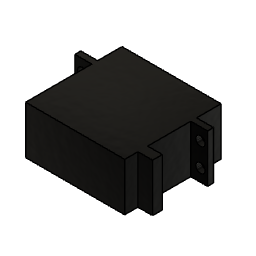
MG995 v10 (Autodesk Fusion 360 design; units mm, degrees)
Autodesk Fusion 360 part; units mm, degrees
sketch "Sketch1" plane through (0, 0, 0) normal (0, 1, 0) x (1, 0, 0)
  line L0 (0, 0) -> (40.47, 0)
  line L1 (40.47, 0) -> (40.47, -39.36)
  line L2 (40.47, -39.36) -> (0, -39.36)
  line L3 (0, -39.36) -> (0, 0)
  line L4 (40.47, -9.96) -> (47.35, -9.96)
  line L5 (47.35, -9.96) -> (47.35, -12.36)
  line L6 (47.35, -12.36) -> (40.47, -12.36)
  line L7 (40.47, -29.96) -> (46.47, -29.96)
  line L8 (46.47, -29.96) -> (46.47, -33.96)
  line L9 (46.47, -33.96) -> (40.47, -33.96)
  line L10 (20.235, 0) -> (20.235, -39.36) construction
  line L11 (0, -9.96) -> (-6.88, -9.96)
  line L12 (-6.88, -9.96) -> (-6.88, -12.36)
  line L13 (-6.88, -12.36) -> (0, -12.36)
  dimension "d1" = 40.47
  dimension "d2" = 39.36
  dimension "d3" = 6.88
  dimension "d4" = 2.4
  dimension "d5" = 27
  dimension "d6" = 6
  dimension "d7" = 4
  dimension "d8" = 5.4
  constraint horizontal L0
  constraint vertical L1
  constraint horizontal L2
  constraint vertical L3
  constraint coincident L0.start L3.end
  constraint coincident L1 L4.start
  constraint perpendicular L1 L4
  constraint perpendicular L4 L5
  constraint coincident L1 L6.end
  constraint perpendicular L1 L6
  constraint horizontal L7
  constraint coincident L1 L7.start
  constraint perpendicular L7 L8
  constraint coincident L1 L9.end
  constraint perpendicular L1 L9
  constraint midpoint L0 L10.start
  constraint midpoint L2 L10.end
  constraint symmetric L4.start L10 L11.start
  constraint symmetric L4.end L10 L11.end
  constraint symmetric L5.end L10 L12.end
  constraint symmetric L6.end L10 L13.end
  measures "d1" distance of L0.start L0.end
  measures "d2" distance of L0.start L2.end
  measures "d3" distance of L4.start L4.end
  measures "d4" distance of L4.end L5.end
  measures "d5" distance of L2 L6
  measures "d6" distance of L7.start L7.end
  measures "d7" distance of L7.end L8.end
  measures "d8" distance of L2 L9
extrude "Extrude1" add sketch "Sketch1" along normal blind 19.6
sketch "Sketch2" plane through (0, 0, 0) normal (0, 0, -1) x (-1, 0, 0)
  line L0 (-40.47, 0) -> (0, 0)
  line L1 (0, 0) -> (0, 19.6)
  line L2 (0, 19.6) -> (-40.47, 19.6)
  line L3 (-40.47, 19.6) -> (-40.47, 0)
  circle A0 centre (-30.8, 9.8) radius 2.92
  line L4 (0, 9.8) -> (-40.47, 9.8) construction
  dimension "d11" = 5.84
  dimension "d12" = 9.67
  constraint midpoint L1 L4.start
  constraint midpoint L3 L4.end
  constraint coincident A0.centre L4
  measures "d11" diameter of A0
  measures "d12" distance of L3 A0.centre
extrude "Extrude2" add sketch "Sketch2" along normal blind 3.81 contours A0
sketch "Sketch3" plane through (0, 0, 9.96) normal (0, 0, -1) x (-1, 0, 0)
  line L0 (-47.35, 0) -> (-40.47, 0)
  line L1 (-40.47, 0) -> (-40.47, 19.6)
  line L2 (-40.47, 19.6) -> (-47.35, 19.6)
  line L3 (-47.35, 19.6) -> (-47.35, 0)
  circle A0 centre (-44.425, 14.58) radius 1.915
  circle A1 centre (-44.425, 5.02) radius 1.915
  line L4 (-40.47, 9.8) -> (-47.35, 9.8) construction
  line L5 (-40.47, 0) -> (-40.47, 19.6)
  line L6 (0, 0) -> (0, 19.6)
  line L7 (0, 0) -> (-40.47, 0)
  line L8 (-40.47, 19.6) -> (0, 19.6)
  line L9 (-20.235, 19.6) -> (-20.235, 0) construction
  dimension "d15" = 3.83
  dimension "d16" = 3.83
  dimension "d17" = 9.56
  dimension "d19" = 2.925
  constraint midpoint L1 L4.start
  constraint midpoint L3 L4.end
  constraint symmetric A0 A1 L4
  constraint midpoint L8 L9.start
  constraint midpoint L7 L9.end
  measures "d15" diameter of A0
  measures "d16" diameter of A1
  measures "d17" distance of A0.centre A1.centre
  measures "d19" distance of L3 A0.centre
extrude "Extrude3" cut sketch "Sketch3" against normal up to surface (2.4 mm away) contours A0 | A1
ref_plane "WorkPlane1" through (20.235, 9.8, 4.98) normal (-1, 0, 0) x (0, 0, 1)
mirror "Mirror1" about plane through (20.235, 9.8, 4.98) normal (-1, 0, 0) of "Extrude3"
